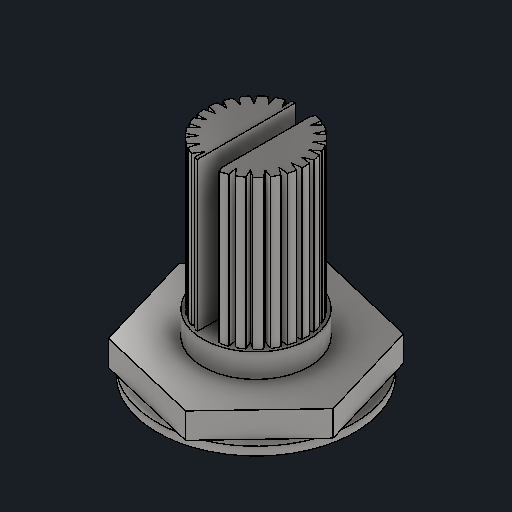
# Autodesk Inventor part: Button_Knob
Saved by Autodesk Inventor 2026.2 (Build 302298000, 298)
## iProperties
Created: 2015-05-06
Part Number: Button_Knob
Material: Stainless Steel
Document SubType Name: Modeling
Designer: Philip
Density: 8 g/cm^3
Appearance: Semi-Polished
Author: Philip
Autodesk Inventor part; units mm, degrees
ref_plane "YZ Plane" through (0, 0, 0) normal (1, 0, 0) x (0, 1, 0)
ref_plane "XZ Plane" through (0, 0, 0) normal (0, 1, 0) x (-1, 0, 0)
ref_plane "XY Plane" through (0, 0, 0) normal (0, 0, 1) x (1, 0, 0)
sketch "Sketch1" plane through (0, 0, 0) normal (0, 1, 0) x (-1, 0, 0)
  circle A0 centre (0, 0) radius 5.9055
  dimension "d0" = 11.811
  constraints: 1 centre point, 1 coincident
  measures "d0" diameter of A0
extrude "Extrusion1" add sketch "Sketch1" along normal blind 0.508
sketch "Sketch2" plane through (0, 0.508, 0) normal (0, 1, 0) x (1, 0, 0)
  line L0 (-6.0608, 1.4528) -> (-1.7723, 5.9752)
  line L1 (-1.7723, 5.9752) -> (4.2885, 4.5224)
  line L2 (4.2885, 4.5224) -> (6.0608, -1.4528)
  line L3 (6.0608, -1.4528) -> (1.7723, -5.9752)
  line L4 (1.7723, -5.9752) -> (-4.2885, -4.5224)
  line L5 (-4.2885, -4.5224) -> (-6.0608, 1.4528)
  point P0 (0, 0)
  point P1 (0, 0)
  dimension "d3" = 10.795
  constraints: 12 end point, 1 coincident, 13 other
  measures "d3" distance between parallel lines of L3 L0
extrude "Extrusion2" add sketch "Sketch2" along normal blind 1.524
sketch "Sketch3" plane through (0, 0, 0) normal (0, -1, 0) x (1, 0, 0)
  circle A0 centre (0, 0) radius 3.175
  dimension "d6" = 6.35
  constraints: 1 centre point, 1 coincident
  measures "d6" diameter of A0
extrude "Extrusion3" add sketch "Sketch3" against normal blind 3.4544
sketch "Sketch4" plane through (0, 3.4544, 0) normal (0, 1, 0) x (1, 0, 0)
  circle A0 centre (0, 0) radius 2.9845
  dimension "d9" = 5.969
  constraints: 1 centre point, 1 coincident
  measures "d9" diameter of A0
extrude "Extrusion4" add sketch "Sketch4" along normal blind 8.89
sketch "Sketch5" plane through (0, 12.3444, 0) normal (0, 1, 0) x (1, 0, 0)
  line L0 (-3.3844, -0.254) -> (-2.4365, 0)
  line L1 (-2.4365, 0) -> (-3.3844, 0.254)
  line L2 (-3.3844, 0.254) -> (-3.3844, -0.254)
  line L3 (0, 0) -> (-2.1237, 0)
  dimension "d12" = 30
  dimension "d13" = 0.508
  dimension "d14" = 0.254
  constraints: 8 end point, 1 horizontal, 1 point on line, 1 vertical
  measures "d12" angle of L1 L0
  measures "d13" distance of L1.end L0.start
  measures "d14" vertical distance of L1.end L0.end
extrude "Extrusion5" cut sketch "Sketch5" against normal blind 8.89
pattern_circular "Circular Pattern2" count 25 over 360 about axis through (0, 3.4544, 0) along (0, 1, 0) of "Extrusion5"
sketch "Sketch6" plane through (0, 12.3444, 0) normal (0, 1, 0) x (1, 0, 0)
  line L0 (0.5715, -4.3158) -> (-0.5715, -4.3158)
  line L1 (-0.5715, -4.3158) -> (-0.5715, 4.3783)
  line L2 (-0.5715, 4.3783) -> (0.5715, 4.3783)
  line L3 (0.5715, 4.3783) -> (0.5715, -4.3158)
  point P0 (0, 0)
  dimension "d23" = 1.143
  dimension "d24" = 0.5715
  constraints: 8 end point, 2 parallel, 1 horizontal, 1 perpendicular
  measures "d23" distance between parallel lines of L3 L1
  measures "d24" distance from line of L1 point (0, 0)
extrude "Extrusion6" cut sketch "Sketch6" against normal blind 8.89
equation "\"d14\" = 0.5 * d13"
equation "\"d24\" = 0.5 * d23"
body "Solid1"
